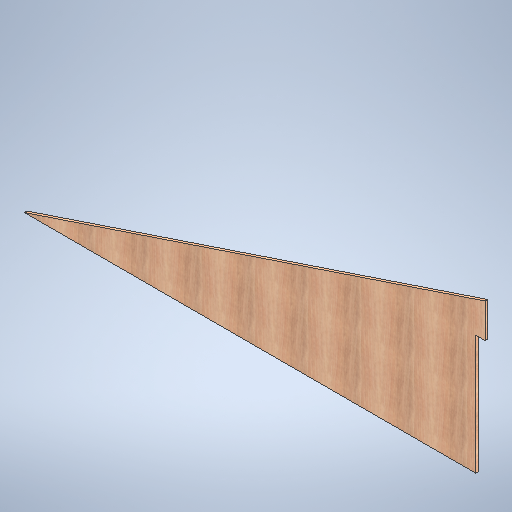
# Autodesk Inventor part: OSB_For_Side_And_Top
Saved by Autodesk Inventor 2025 (Build 290162010, 162A)
## iProperties
Created: 2024-09-19
Part Number: OSB_For_Side_And_Top
Material: Wood (Birch)
Document SubType Name: Modeling
Designer: Tom
Density: 0.55 g/cm^3
Appearance: Birch - Natural Polished
Author: Tom
Autodesk Inventor part; units mm, degrees
ref_plane "YZ Plane" through (0, 0, 0) normal (1, 0, 0) x (0, 1, 0)
ref_plane "XZ Plane" through (0, 0, 0) normal (0, 1, 0) x (-1, 0, 0)
ref_plane "XY Plane" through (0, 0, 0) normal (0, 0, 1) x (1, 0, 0)
sketch "Sketch1" plane through (0, 0, 0) normal (0, 0, 1) x (1, 0, 0)
  line L0 (0, 0) -> (0, 758.1646)
  line L1 (0, 0) -> (1219.2, 0)
  line L2 (0, 758.1646) -> (3365.5, 1881.0892)
  line L3 (12.7, 762.4021) -> (12.7, 0)
  line L4 (3365.5, 1881.0892) -> (3365.5, 1733.8182)
  line L5 (3365.5, 1733.8182) -> (101.6, 644.7932)
  line L6 (101.6, 644.7932) -> (12.7, 644.7932)
  line L7 (1219.2, 0) -> (1219.2, 1164.9599)
  line L8 (0, 758.1646) -> (-35.0901, 746.4565)
  line L9 (-35.0901, 746.4565) -> (-35.0901, 644.7932)
  line L10 (-35.0901, 644.7932) -> (0, 644.7932)
  line L11 (-35.0901, 746.4565) -> (-40.1146, 761.5154)
  line L12 (-40.1146, 761.5154) -> (1219.2, 1181.6953)
  line L13 (1219.2, 1181.6953) -> (1219.2, 1164.9599)
  line L14 (1219.2, 1181.6953) -> (3378.2, 1181.6953)
  line L15 (3378.2, 1181.6953) -> (3378.2, 0)
  line L16 (3378.2, 0) -> (1219.2, 0)
  line L17 (3365.5, 1881.0892) -> (3422.8151, 1900.2128)
  line L18 (3422.8151, 1900.2128) -> (3422.8151, 1752.9418)
  line L19 (3365.5, 1733.8182) -> (3422.8151, 1752.9418)
  line L20 (3422.8151, 1752.9418) -> (3365.5, 1752.9418)
  line L21 (1219.2, 1181.6953) -> (3422.8151, 1916.9482)
  line L22 (3422.8151, 1916.9482) -> (3422.8151, 1900.2128)
  line L23 (3378.2, 1181.6953) -> (3378.2, 1752.9418)
  line L24 (3378.2, 1752.9418) -> (3422.8151, 1752.9418)
  line L25 (3422.8151, 1752.9418) -> (3422.8151, 1900.2128)
  dimension "d1" = 758.1646
  dimension "d3" = 12.7
  dimension "d4" = 3352.8
  dimension "d6" = 139.7
  dimension "d8" = 88.9
  dimension "d9" = 1089.025
  dimension "d12" = 47.7901
  dimension "d14" = 15.875
  dimension "d16" = 1219.2
  dimension "d17" = 2159
  dimension "d20" = 57.3151
  constraints: 52 end point, 8 collinear, 8 vertical, 7 point on line, 5 horizontal, 3 parallel, 2 perpendicular
  measures "d1" distance of L0.start L0.end
  measures "d3" distance between parallel lines of L3 L0
  measures "d4" distance from line of L3 L2.end
  measures "d6" distance between parallel lines of L2 L5
  measures "d8" horizontal distance of L3.start L5.end
  measures "d9" vertical distance of L4.end L5.end
  measures "d12" distance between parallel lines of L9 L3
  measures "d14" distance between parallel lines of L2 L12
  measures "d16" distance of L0.start L1.end
  measures "d17" distance of L15.end L1.end
  measures "d20" distance between parallel lines of L18 L4
extrude "Extrusion1" add sketch "Sketch1" along normal blind 12.7 contours L14 L2 L4 L5 | L5 L19 L23 L14 | L14 L21 L22 L17 L2 | L4 L20 L23 L19 | L17 L18 L20 L4
body "Solid1"
